Autodesk Inventor part; units mm, degrees
(part 2 of 3)
  line L384 (86.5601, -24.0434) -> (86.5601, -7.2718)
  line L385 (91.5601, -7.2718) -> (91.5601, -24.0434)
  arc A154 (86.853, -6.5647) -> (86.5601, -7.2718) centre (87.5601, -7.2718) ccw
  line L386 (86.853, -6.5647) -> (88.7601, -4.6576)
  line L387 (89.0601, -4.6576) -> (88.7601, -4.6576)
  line L388 (89.0601, -4.6576) -> (89.3601, -4.6576)
  arc A155 (91.5601, -7.2718) -> (91.2672, -6.5647) centre (90.5601, -7.2718) ccw
  line L389 (91.2672, -6.5647) -> (89.3601, -4.6576)
  arc A156 (116.0672, 0.0495) -> (116.3601, 0.7566) centre (115.3601, 0.7566) ccw
  arc A157 (111.3601, 0.7566) -> (111.653, 0.0495) centre (112.3601, 0.7566) ccw
  line L390 (116.0672, 0.0495) -> (114.1601, -1.8576)
  line L391 (111.653, 0.0495) -> (113.5601, -1.8576)
  line L392 (113.8601, -1.8576) -> (114.1601, -1.8576)
  line L393 (113.8601, -1.8576) -> (113.5601, -1.8576)
  line L394 (111.3601, 0.7566) -> (111.3601, 17.5282)
  line L395 (116.3601, 17.5282) -> (116.3601, 0.7566)
  arc A158 (111.653, 18.2353) -> (111.3601, 17.5282) centre (112.3601, 17.5282) ccw
  line L396 (111.653, 18.2353) -> (113.5601, 20.1424)
  line L397 (113.8601, 20.1424) -> (113.5601, 20.1424)
  line L398 (113.8601, 20.1424) -> (114.1601, 20.1424)
  arc A159 (116.3601, 17.5282) -> (116.0672, 18.2353) centre (115.3601, 17.5282) ccw
  line L399 (116.0672, 18.2353) -> (114.1601, 20.1424)
  arc A160 (116.0672, -24.7505) -> (116.3601, -24.0434) centre (115.3601, -24.0434) ccw
  arc A161 (111.3601, -24.0434) -> (111.653, -24.7505) centre (112.3601, -24.0434) ccw
  line L400 (116.0672, -24.7505) -> (114.1601, -26.6576)
  line L401 (111.653, -24.7505) -> (113.5601, -26.6576)
  line L402 (113.8601, -26.6576) -> (114.1601, -26.6576)
  line L403 (113.8601, -26.6576) -> (113.5601, -26.6576)
  line L404 (111.3601, -24.0434) -> (111.3601, -7.2718)
  line L405 (116.3601, -7.2718) -> (116.3601, -24.0434)
  arc A162 (111.653, -6.5647) -> (111.3601, -7.2718) centre (112.3601, -7.2718) ccw
  line L406 (111.653, -6.5647) -> (113.5601, -4.6576)
  line L407 (113.8601, -4.6576) -> (113.5601, -4.6576)
  line L408 (113.8601, -4.6576) -> (114.1601, -4.6576)
  arc A163 (116.3601, -7.2718) -> (116.0672, -6.5647) centre (115.3601, -7.2718) ccw
  line L409 (116.0672, -6.5647) -> (114.1601, -4.6576)
  arc A164 (92.3672, -30.2647) -> (93.0743, -30.5576) centre (93.0743, -29.5576) ccw
  arc A165 (93.0743, -25.5576) -> (92.3672, -25.8505) centre (93.0743, -26.5576) ccw
  line L410 (92.3672, -30.2647) -> (90.4601, -28.3576)
  line L411 (92.3672, -25.8505) -> (90.4601, -27.7576)
  line L412 (90.4601, -28.0576) -> (90.4601, -28.3576)
  line L413 (90.4601, -28.0576) -> (90.4601, -27.7576)
  line L414 (93.0743, -25.5576) -> (109.8459, -25.5576)
  line L415 (109.8459, -30.5576) -> (93.0743, -30.5576)
  arc A166 (110.553, -25.8505) -> (109.8459, -25.5576) centre (109.8459, -26.5576) ccw
  line L416 (110.553, -25.8505) -> (112.4601, -27.7576)
  line L417 (112.4601, -28.0576) -> (112.4601, -27.7576)
  line L418 (112.4601, -28.0576) -> (112.4601, -28.3576)
  arc A167 (109.8459, -30.5576) -> (110.553, -30.2647) centre (109.8459, -29.5576) ccw
  line L419 (110.553, -30.2647) -> (112.4601, -28.3576)
  line L420 (-43.8399, 8.0424) -> (-42.8399, 8.0424)
  line L421 (-42.8399, 8.0424) -> (-40.8399, 6.0424)
  line L422 (-40.8399, 6.0424) -> (-40.8399, 5.0424)
  line L423 (-40.8399, 5.0424) -> (-42.8399, 3.0424)
  line L424 (-42.8399, 3.0424) -> (-43.8399, 3.0424)
  line L425 (-43.8399, 3.0424) -> (-45.8399, 5.0424)
  line L426 (-45.8399, 5.0424) -> (-45.8399, 6.0424)
  line L427 (-45.8399, 6.0424) -> (-43.8399, 8.0424)
  line L428 (-43.8399, -11.9576) -> (-42.8399, -11.9576)
  line L429 (-42.8399, -11.9576) -> (-40.8399, -13.9576)
  line L430 (-40.8399, -13.9576) -> (-40.8399, -14.9576)
  line L431 (-40.8399, -14.9576) -> (-42.8399, -16.9576)
  line L432 (-42.8399, -16.9576) -> (-43.8399, -16.9576)
  line L433 (-43.8399, -16.9576) -> (-45.8399, -14.9576)
  line L434 (-45.8399, -14.9576) -> (-45.8399, -13.9576)
  line L435 (-45.8399, -13.9576) -> (-43.8399, -11.9576)
  line L436 (40.2601, 8.0424) -> (41.2601, 8.0424)
  line L437 (41.2601, 8.0424) -> (43.2601, 6.0424)
  line L438 (43.2601, 6.0424) -> (43.2601, 5.0424)
  line L439 (43.2601, 5.0424) -> (41.2601, 3.0424)
  line L440 (41.2601, 3.0424) -> (40.2601, 3.0424)
  line L441 (40.2601, 3.0424) -> (38.2601, 5.0424)
  line L442 (38.2601, 5.0424) -> (38.2601, 6.0424)
  line L443 (38.2601, 6.0424) -> (40.2601, 8.0424)
  line L444 (40.2601, -11.9576) -> (41.2601, -11.9576)
  line L445 (41.2601, -11.9576) -> (43.2601, -13.9576)
  line L446 (43.2601, -13.9576) -> (43.2601, -14.9576)
  line L447 (43.2601, -14.9576) -> (41.2601, -16.9576)
  line L448 (41.2601, -16.9576) -> (40.2601, -16.9576)
  line L449 (40.2601, -16.9576) -> (38.2601, -14.9576)
  line L450 (38.2601, -14.9576) -> (38.2601, -13.9576)
  line L451 (38.2601, -13.9576) -> (40.2601, -11.9576)
  arc A168 (-141.5328, -5.6647) -> (-140.8257, -5.9576) centre (-140.8257, -4.9576) ccw
  arc A169 (-140.8257, -0.9576) -> (-141.5328, -1.2505) centre (-140.8257, -1.9576) ccw
  line L452 (-141.5328, -5.6647) -> (-143.4399, -3.7576)
  line L453 (-143.4399, -3.4576) -> (-143.4399, -3.1576)
  line L454 (-143.4399, -3.4576) -> (-143.4399, -3.7576)
  line L455 (-141.5328, -1.2505) -> (-143.4399, -3.1576)
  line L456 (-140.8257, -0.9576) -> (-130.0541, -0.9576)
  line L457 (-130.0541, -5.9576) -> (-140.8257, -5.9576)
  arc A170 (-129.347, -1.2505) -> (-130.0541, -0.9576) centre (-130.0541, -1.9576) ccw
  arc A171 (-130.0541, -5.9576) -> (-129.347, -5.6647) centre (-130.0541, -4.9576) ccw
  line L458 (-129.347, -5.6647) -> (-127.4399, -3.7576)
  line L459 (-127.4399, -3.4576) -> (-127.4399, -3.7576)
  line L460 (-127.4399, -3.4576) -> (-127.4399, -3.1576)
  line L461 (-129.347, -1.2505) -> (-127.4399, -3.1576)
  arc A172 (-142.2328, -0.5505) -> (-141.9399, 0.1566) centre (-142.9399, 0.1566) ccw
  arc A173 (-146.9399, 0.1566) -> (-146.647, -0.5505) centre (-145.9399, 0.1566) ccw
  line L462 (-142.2328, -0.5505) -> (-144.1399, -2.4576)
  line L463 (-144.4399, -2.4576) -> (-144.7399, -2.4576)
  line L464 (-144.4399, -2.4576) -> (-144.1399, -2.4576)
  line L465 (-146.647, -0.5505) -> (-144.7399, -2.4576)
  line L466 (-146.9399, 0.1566) -> (-146.9399, 10.9282)
  line L467 (-141.9399, 10.9282) -> (-141.9399, 0.1566)
  arc A174 (-146.647, 11.6353) -> (-146.9399, 10.9282) centre (-145.9399, 10.9282) ccw
  arc A175 (-141.9399, 10.9282) -> (-142.2328, 11.6353) centre (-142.9399, 10.9282) ccw
  line L468 (-142.2328, 11.6353) -> (-144.1399, 13.5424)
  line L469 (-144.4399, 13.5424) -> (-144.1399, 13.5424)
  line L470 (-144.4399, 13.5424) -> (-144.7399, 13.5424)
  line L471 (-146.647, 11.6353) -> (-144.7399, 13.5424)
  arc A176 (-159.5328, -5.6647) -> (-158.8257, -5.9576) centre (-158.8257, -4.9576) ccw
  arc A177 (-158.8257, -0.9576) -> (-159.5328, -1.2505) centre (-158.8257, -1.9576) ccw
  line L472 (-159.5328, -5.6647) -> (-161.4399, -3.7576)
  line L473 (-161.4399, -3.4576) -> (-161.4399, -3.1576)
  line L474 (-161.4399, -3.4576) -> (-161.4399, -3.7576)
  line L475 (-159.5328, -1.2505) -> (-161.4399, -3.1576)
  line L476 (-158.8257, -0.9576) -> (-148.0541, -0.9576)
  line L477 (-148.0541, -5.9576) -> (-158.8257, -5.9576)
  arc A178 (-147.347, -1.2505) -> (-148.0541, -0.9576) centre (-148.0541, -1.9576) ccw
  arc A179 (-148.0541, -5.9576) -> (-147.347, -5.6647) centre (-148.0541, -4.9576) ccw
  line L478 (-147.347, -5.6647) -> (-145.4399, -3.7576)
  line L479 (-145.4399, -3.4576) -> (-145.4399, -3.7576)
  line L480 (-145.4399, -3.4576) -> (-145.4399, -3.1576)
  line L481 (-147.347, -1.2505) -> (-145.4399, -3.1576)
  arc A180 (-142.2328, -18.5505) -> (-141.9399, -17.8434) centre (-142.9399, -17.8434) ccw
  arc A181 (-146.9399, -17.8434) -> (-146.647, -18.5505) centre (-145.9399, -17.8434) ccw
  line L482 (-142.2328, -18.5505) -> (-144.1399, -20.4576)
  line L483 (-144.4399, -20.4576) -> (-144.7399, -20.4576)
  line L484 (-144.4399, -20.4576) -> (-144.1399, -20.4576)
  line L485 (-146.647, -18.5505) -> (-144.7399, -20.4576)
  line L486 (-146.9399, -17.8434) -> (-146.9399, -7.0718)
  line L487 (-141.9399, -7.0718) -> (-141.9399, -17.8434)
  arc A182 (-146.647, -6.3647) -> (-146.9399, -7.0718) centre (-145.9399, -7.0718) ccw
  arc A183 (-141.9399, -7.0718) -> (-142.2328, -6.3647) centre (-142.9399, -7.0718) ccw
  line L488 (-142.2328, -6.3647) -> (-144.1399, -4.4576)
  line L489 (-144.4399, -4.4576) -> (-144.1399, -4.4576)
  line L490 (-144.4399, -4.4576) -> (-144.7399, -4.4576)
  line L491 (-146.647, -6.3647) -> (-144.7399, -4.4576)
  arc A184 (-170.0328, 10.3353) -> (-169.3257, 10.0424) centre (-169.3257, 11.0424) ccw
  arc A185 (-169.3257, 15.0424) -> (-170.0328, 14.7495) centre (-169.3257, 14.0424) ccw
  line L492 (-170.0328, 10.3353) -> (-171.9399, 12.2424)
  line L493 (-171.9399, 12.5424) -> (-171.9399, 12.8424)
  line L494 (-171.9399, 12.5424) -> (-171.9399, 12.2424)
  line L495 (-170.0328, 14.7495) -> (-171.9399, 12.8424)
  line L496 (-169.3257, 15.0424) -> (-158.5541, 15.0424)
  line L497 (-158.5541, 10.0424) -> (-169.3257, 10.0424)
  arc A186 (-157.847, 14.7495) -> (-158.5541, 15.0424) centre (-158.5541, 14.0424) ccw
  arc A187 (-158.5541, 10.0424) -> (-157.847, 10.3353) centre (-158.5541, 11.0424) ccw
  line L498 (-157.847, 10.3353) -> (-155.9399, 12.2424)
  line L499 (-155.9399, 12.5424) -> (-155.9399, 12.2424)
  line L500 (-155.9399, 12.5424) -> (-155.9399, 12.8424)
  line L501 (-157.847, 14.7495) -> (-155.9399, 12.8424)
  arc A188 (-187.0328, 10.3353) -> (-186.3257, 10.0424) centre (-186.3257, 11.0424) ccw
  arc A189 (-186.3257, 15.0424) -> (-187.0328, 14.7495) centre (-186.3257, 14.0424) ccw
  line L502 (-187.0328, 10.3353) -> (-188.9399, 12.2424)
  line L503 (-188.9399, 12.5424) -> (-188.9399, 12.8424)
  line L504 (-188.9399, 12.5424) -> (-188.9399, 12.2424)
  line L505 (-187.0328, 14.7495) -> (-188.9399, 12.8424)
  line L506 (-186.3257, 15.0424) -> (-175.5541, 15.0424)
  line L507 (-175.5541, 10.0424) -> (-186.3257, 10.0424)
  arc A190 (-174.847, 14.7495) -> (-175.5541, 15.0424) centre (-175.5541, 14.0424) ccw
  arc A191 (-175.5541, 10.0424) -> (-174.847, 10.3353) centre (-175.5541, 11.0424) ccw
  line L508 (-174.847, 10.3353) -> (-172.9399, 12.2424)
  line L509 (-172.9399, 12.5424) -> (-172.9399, 12.2424)
  line L510 (-172.9399, 12.5424) -> (-172.9399, 12.8424)
  line L511 (-174.847, 14.7495) -> (-172.9399, 12.8424)
  arc A192 (-170.2328, -3.0647) -> (-169.9399, -2.3576) centre (-170.9399, -2.3576) ccw
  arc A193 (-174.9399, -2.3576) -> (-174.647, -3.0647) centre (-173.9399, -2.3576) ccw
  line L512 (-170.2328, -3.0647) -> (-172.1399, -4.9718)
  line L513 (-172.4399, -4.9718) -> (-172.7399, -4.9718)
  line L514 (-172.4399, -4.9718) -> (-172.1399, -4.9718)
  line L515 (-174.647, -3.0647) -> (-172.7399, -4.9718)
  line L516 (-174.9399, -2.3576) -> (-174.9399, 8.414)
  line L517 (-169.9399, 8.414) -> (-169.9399, -2.3576)
  arc A194 (-174.647, 9.1211) -> (-174.9399, 8.414) centre (-173.9399, 8.414) ccw
  arc A195 (-169.9399, 8.414) -> (-170.2328, 9.1211) centre (-170.9399, 8.414) ccw
  line L518 (-170.2328, 9.1211) -> (-172.1399, 11.0282)
  line L519 (-172.4399, 11.0282) -> (-172.1399, 11.0282)
  line L520 (-172.4399, 11.0282) -> (-172.7399, 11.0282)
  line L521 (-174.647, 9.1211) -> (-172.7399, 11.0282)
  arc A196 (-170.2328, -19.5647) -> (-169.9399, -18.8576) centre (-170.9399, -18.8576) ccw
  arc A197 (-174.9399, -18.8576) -> (-174.647, -19.5647) centre (-173.9399, -18.8576) ccw
  line L522 (-170.2328, -19.5647) -> (-172.1399, -21.4718)
  line L523 (-172.4399, -21.4718) -> (-172.7399, -21.4718)
  line L524 (-172.4399, -21.4718) -> (-172.1399, -21.4718)
  line L525 (-174.647, -19.5647) -> (-172.7399, -21.4718)
  line L526 (-174.9399, -18.8576) -> (-174.9399, -8.086)
  line L527 (-169.9399, -8.086) -> (-169.9399, -18.8576)
  arc A198 (-174.647, -7.3789) -> (-174.9399, -8.086) centre (-173.9399, -8.086) ccw
  arc A199 (-169.9399, -8.086) -> (-170.2328, -7.3789) centre (-170.9399, -8.086) ccw
  line L528 (-170.2328, -7.3789) -> (-172.1399, -5.4718)
  line L529 (-172.4399, -5.4718) -> (-172.1399, -5.4718)
  line L530 (-172.4399, -5.4718) -> (-172.7399, -5.4718)
  line L531 (-174.647, -7.3789) -> (-172.7399, -5.4718)
  point P0 (-22.4267, -1.12)
  dimension "d362" = 7.5
  dimension "d363" = 17
  dimension "d364" = 7.5
  dimension "d365" = 17
  dimension "d366" = 7.5
  dimension "d367" = 0
  dimension "d368" = 0
  dimension "d369" = 0
  dimension "d370" = 0
  dimension "d371" = 0
  dimension "d372" = 15
  dimension "d373" = 0
  dimension "d374" = 16
  dimension "d375" = 6
  dimension "d376" = 6
  dimension "d377" = 13.6
  dimension "d378" = 16
  dimension "d379" = 6
  dimension "d380" = 15
  dimension "d381" = 0
  dimension "d509" = 23
  dimension "d510" = 25
  dimension "d511" = 24.6
  dimension "d514" = 0.5
sketch "Clock Front Face Outline" plane through (0, 0, 0) normal (0, 0, 1) x (1, 0, 0)
  line L0 (-365.1075, -11.3808) -> (-85.1075, -11.3808)
  line L1 (-60.1075, -36.3808) -> (-60.1075, -56.3808)
  line L2 (-85.1075, -81.3808) -> (-365.1075, -81.3808)
  line L3 (-390.1075, -56.3808) -> (-390.1075, -36.3808)
  arc A0 (-365.1075, -11.3808) -> (-390.1075, -36.3808) centre (-365.1075, -36.3808) ccw
  arc A1 (-60.1075, -36.3808) -> (-85.1075, -11.3808) centre (-85.1075, -36.3808) ccw
  arc A2 (-85.1075, -81.3808) -> (-60.1075, -56.3808) centre (-85.1075, -56.3808) ccw
  arc A3 (-390.1075, -56.3808) -> (-365.1075, -81.3808) centre (-365.1075, -56.3808) ccw
  point P0 (0, -2.2581)
  dimension "d429" = 330
  dimension "d430" = 70
  dimension "d431" = 25
  measures "d429" distance between parallel lines of L1 L3
  measures "d430" distance between parallel lines of L2 L0
  measures "d431" radius of A0
sketch "Small Segmemt" plane through (0, 0, 0) normal (0, 0, 1) x (1, 0, 0)
  arc A0 (-247.3536, -9.433) -> (-246.6465, -9.7259) centre (-246.6465, -8.7259) ccw
  arc A1 (-246.6465, -4.7259) -> (-247.3536, -5.0187) centre (-246.6465, -5.7259) ccw
  line L0 (-247.3536, -9.433) -> (-249.2607, -7.5259)
  line L1 (-249.2607, -7.2259) -> (-249.2607, -6.9259)
  line L2 (-249.2607, -7.2259) -> (-249.2607, -7.5259)
  line L3 (-247.3536, -5.0187) -> (-249.2607, -6.9259)
  line L4 (-246.6465, -4.7259) -> (-235.875, -4.7259)
  line L5 (-235.875, -9.7259) -> (-246.6465, -9.7259)
  arc A2 (-235.1679, -5.0187) -> (-235.875, -4.7259) centre (-235.875, -5.7259) ccw
  arc A3 (-235.875, -9.7259) -> (-235.1679, -9.433) centre (-235.875, -8.7259) ccw
  line L6 (-235.1679, -9.433) -> (-233.2607, -7.5259)
  line L7 (-233.2607, -7.2259) -> (-233.2607, -7.5259)
  line L8 (-233.2607, -7.2259) -> (-233.2607, -6.9259)
  line L9 (-235.1679, -5.0187) -> (-233.2607, -6.9259)
  point P0 (-225.4266, -6.7349)
  point P1 (-247.0607, -4.7259)
  point P2 (-247.0607, -9.7259)
  point P3 (-235.4607, -4.7259)
  point P4 (-235.4607, -9.7259)
  dimension "d462" = 2.2
  dimension "d463" = 2.2
  dimension "d464" = 2.2
  dimension "d465" = 2.2
  dimension "d466" = 2.2
  dimension "d467" = 2.2
  dimension "d468" = 2.2
  dimension "d469" = 1
  dimension "d470" = 5
  dimension "d471" = 2.2
  dimension "d472" = 2.2
  dimension "d473" = 135
  dimension "d474" = 16
  dimension "d475" = 135
  dimension "d476" = 2.5
  dimension "d477" = 5
  dimension "d478" = 16
  dimension "d479" = 2.2
  dimension "d480" = 0.3
  dimension "d481" = 0.3
  dimension "d482" = 0.3
  dimension "d483" = 0.3
  measures "d462" horizontal distance of point (-247.061, -9.726) L0.end
  measures "d463" horizontal distance of L8.end point (-235.461, -4.726)
  measures "d464" horizontal distance of point (-247.061, -4.726) L1.end
  measures "d465" horizontal distance of L6.end point (-235.461, -9.726)
  measures "d466" horizontal distance of L6.end point (-235.461, -9.726)
  measures "d467" horizontal distance of point (-247.061, -4.726) L1.end
  measures "d468" horizontal distance of point (-247.061, -9.726) L0.end
  measures "d469" radius of A1
  measures "d470" distance of point (-235.461, -9.726) point (-235.461, -4.726)
  measures "d471" horizontal distance of L8.end point (-235.461, -4.726)
  measures "d472" horizontal distance of point (-235.461, -9.726) L7.start
  measures "d473" angle of L5 L6
  measures "d474" horizontal distance of L6.end L1.start
  measures "d475" angle of L4 L9
  measures "d476" vertical distance of L7.start point (-235.461, -9.726)
  measures "d477" distance between parallel lines of L5 L4
  measures "d478" distance of L1.start L7.start
  measures "d479" horizontal distance of point (-247.061, -4.726) L1.start
  measures "d480" distance of L7.start L8.end
  measures "d481" distance of L6.end L7.start
  measures "d482" distance of L1.end L1.start
  measures "d483" distance of L0.end L1.start
sketch "Sketch1" plane through (0, 0, 0) normal (0, 0, 1) x (1, 0, 0)
  line L0 (-365.1075, -11.3808) -> (-85.1075, -11.3808)
  line L1 (-60.1075, -36.3808) -> (-60.1075, -56.3808)
  line L2 (-85.1075, -81.3808) -> (-365.1075, -81.3808)
  line L3 (-390.1075, -56.3808) -> (-390.1075, -36.3808)
  arc A0 (-365.1075, -11.3808) -> (-390.1075, -36.3808) centre (-365.1075, -36.3808) ccw
  arc A1 (-60.1075, -36.3808) -> (-85.1075, -11.3808) centre (-85.1075, -36.3808) ccw
  arc A2 (-85.1075, -81.3808) -> (-60.1075, -56.3808) centre (-85.1075, -56.3808) ccw
  arc A3 (-390.1075, -56.3808) -> (-365.1075, -81.3808) centre (-365.1075, -56.3808) ccw
  point P0 (0, 0)
extrude "Extrusion1" add sketch "Sketch1" along normal blind 3
sketch "Sketch5" plane through (0, 0, 3) normal (0, 0, 1) x (1, 0, 0)
  line L0 (-85.1075, -11.3808) -> (-365.1075, -11.3808) projected
  line L1 (-365.1075, -81.3808) -> (-85.1075, -81.3808) projected
  line L2 (-390.1075, -36.3808) -> (-390.1075, -56.3808) projected
  line L3 (-60.1075, -56.3808) -> (-60.1075, -36.3808) projected
  arc A0 (-138.1004, -24.0879) -> (-137.3933, -24.3808) centre (-137.3933, -23.3808) ccw
  arc A1 (-137.3933, -19.3808) -> (-138.1004, -19.6736) centre (-137.3933, -20.3808) ccw
  line L4 (-138.1004, -24.0879) -> (-140.0075, -22.1808)
  line L5 (-138.1004, -19.6736) -> (-140.0075, -21.5808)
  line L6 (-140.0075, -21.8808) -> (-140.0075, -22.1808)
  line L7 (-140.0075, -21.8808) -> (-140.0075, -21.5808)
  line L8 (-137.3933, -19.3808) -> (-120.6217, -19.3808)
  line L9 (-120.6217, -24.3808) -> (-137.3933, -24.3808)
  arc A2 (-119.9146, -19.6736) -> (-120.6217, -19.3808) centre (-120.6217, -20.3808) ccw
  line L10 (-119.9146, -19.6736) -> (-118.0075, -21.5808)
  line L11 (-118.0075, -21.8808) -> (-118.0075, -21.5808)
  line L12 (-118.0075, -21.8808) -> (-118.0075, -22.1808)
  arc A3 (-120.6217, -24.3808) -> (-119.9146, -24.0879) centre (-120.6217, -23.3808) ccw
  line L13 (-119.9146, -24.0879) -> (-118.0075, -22.1808)
  arc A4 (-138.1004, -48.8879) -> (-137.3933, -49.1808) centre (-137.3933, -48.1808) ccw
  arc A5 (-137.3933, -44.1808) -> (-138.1004, -44.4736) centre (-137.3933, -45.1808) ccw
  line L14 (-138.1004, -48.8879) -> (-140.0075, -46.9808)
  line L15 (-138.1004, -44.4736) -> (-140.0075, -46.3808)
  line L16 (-140.0075, -46.6808) -> (-140.0075, -46.9808)
  line L17 (-140.0075, -46.6808) -> (-140.0075, -46.3808)
  line L18 (-137.3933, -44.1808) -> (-120.6217, -44.1808)
  line L19 (-120.6217, -49.1808) -> (-137.3933, -49.1808)
  arc A6 (-119.9146, -44.4736) -> (-120.6217, -44.1808) centre (-120.6217, -45.1808) ccw
  line L20 (-119.9146, -44.4736) -> (-118.0075, -46.3808)
  line L21 (-118.0075, -46.6808) -> (-118.0075, -46.3808)
  line L22 (-118.0075, -46.6808) -> (-118.0075, -46.9808)
  arc A7 (-120.6217, -49.1808) -> (-119.9146, -48.8879) centre (-120.6217, -48.1808) ccw
  line L23 (-119.9146, -48.8879) -> (-118.0075, -46.9808)
  arc A8 (-139.2004, -43.3736) -> (-138.9075, -42.6665) centre (-139.9075, -42.6665) ccw
  arc A9 (-143.9075, -42.6665) -> (-143.6146, -43.3736) centre (-142.9075, -42.6665) ccw
  line L24 (-139.2004, -43.3736) -> (-141.1075, -45.2808)
  line L25 (-143.6146, -43.3736) -> (-141.7075, -45.2808)
  line L26 (-141.4075, -45.2808) -> (-141.1075, -45.2808)
  line L27 (-141.4075, -45.2808) -> (-141.7075, -45.2808)
  line L28 (-143.9075, -42.6665) -> (-143.9075, -25.895)
  line L29 (-138.9075, -25.895) -> (-138.9075, -42.6665)
  arc A10 (-143.6146, -25.1879) -> (-143.9075, -25.895) centre (-142.9075, -25.895) ccw
  line L30 (-143.6146, -25.1879) -> (-141.7075, -23.2808)
  line L31 (-141.4075, -23.2808) -> (-141.7075, -23.2808)
  line L32 (-141.4075, -23.2808) -> (-141.1075, -23.2808)
  arc A11 (-138.9075, -25.895) -> (-139.2004, -25.1879) centre (-139.9075, -25.895) ccw
  line L33 (-139.2004, -25.1879) -> (-141.1075, -23.2808)
  arc A12 (-139.2004, -68.1736) -> (-138.9075, -67.4665) centre (-139.9075, -67.4665) ccw
  arc A13 (-143.9075, -67.4665) -> (-143.6146, -68.1736) centre (-142.9075, -67.4665) ccw
  line L34 (-139.2004, -68.1736) -> (-141.1075, -70.0808)
  line L35 (-143.6146, -68.1736) -> (-141.7075, -70.0808)
  line L36 (-141.4075, -70.0808) -> (-141.1075, -70.0808)
  line L37 (-141.4075, -70.0808) -> (-141.7075, -70.0808)
  line L38 (-143.9075, -67.4665) -> (-143.9075, -50.695)
  line L39 (-138.9075, -50.695) -> (-138.9075, -67.4665)
  arc A14 (-143.6146, -49.9879) -> (-143.9075, -50.695) centre (-142.9075, -50.695) ccw
  line L40 (-143.6146, -49.9879) -> (-141.7075, -48.0808)
  line L41 (-141.4075, -48.0808) -> (-141.7075, -48.0808)
  line L42 (-141.4075, -48.0808) -> (-141.1075, -48.0808)
  arc A15 (-138.9075, -50.695) -> (-139.2004, -49.9879) centre (-139.9075, -50.695) ccw
  line L43 (-139.2004, -49.9879) -> (-141.1075, -48.0808)
  arc A16 (-114.4004, -43.3736) -> (-114.1075, -42.6665) centre (-115.1075, -42.6665) ccw
  arc A17 (-119.1075, -42.6665) -> (-118.8146, -43.3736) centre (-118.1075, -42.6665) ccw
  line L44 (-114.4004, -43.3736) -> (-116.3075, -45.2808)
  line L45 (-118.8146, -43.3736) -> (-116.9075, -45.2808)
  line L46 (-116.6075, -45.2808) -> (-116.3075, -45.2808)
  line L47 (-116.6075, -45.2808) -> (-116.9075, -45.2808)
  line L48 (-119.1075, -42.6665) -> (-119.1075, -25.895)
  line L49 (-114.1075, -25.895) -> (-114.1075, -42.6665)
  arc A18 (-118.8146, -25.1879) -> (-119.1075, -25.895) centre (-118.1075, -25.895) ccw
  line L50 (-118.8146, -25.1879) -> (-116.9075, -23.2808)
  line L51 (-116.6075, -23.2808) -> (-116.9075, -23.2808)
  line L52 (-116.6075, -23.2808) -> (-116.3075, -23.2808)
  arc A19 (-114.1075, -25.895) -> (-114.4004, -25.1879) centre (-115.1075, -25.895) ccw
  line L53 (-114.4004, -25.1879) -> (-116.3075, -23.2808)
  arc A20 (-114.4004, -68.1736) -> (-114.1075, -67.4665) centre (-115.1075, -67.4665) ccw
  arc A21 (-119.1075, -67.4665) -> (-118.8146, -68.1736) centre (-118.1075, -67.4665) ccw
  line L54 (-114.4004, -68.1736) -> (-116.3075, -70.0808)
  line L55 (-118.8146, -68.1736) -> (-116.9075, -70.0808)
  line L56 (-116.6075, -70.0808) -> (-116.3075, -70.0808)
  line L57 (-116.6075, -70.0808) -> (-116.9075, -70.0808)
  line L58 (-119.1075, -67.4665) -> (-119.1075, -50.695)
  line L59 (-114.1075, -50.695) -> (-114.1075, -67.4665)
  arc A22 (-118.8146, -49.9879) -> (-119.1075, -50.695) centre (-118.1075, -50.695) ccw
  line L60 (-118.8146, -49.9879) -> (-116.9075, -48.0808)
  line L61 (-116.6075, -48.0808) -> (-116.9075, -48.0808)
  line L62 (-116.6075, -48.0808) -> (-116.3075, -48.0808)
  arc A23 (-114.1075, -50.695) -> (-114.4004, -49.9879) centre (-115.1075, -50.695) ccw
  line L63 (-114.4004, -49.9879) -> (-116.3075, -48.0808)
  arc A24 (-138.1004, -73.6879) -> (-137.3933, -73.9808) centre (-137.3933, -72.9808) ccw
  arc A25 (-137.3933, -68.9808) -> (-138.1004, -69.2736) centre (-137.3933, -69.9808) ccw
  line L64 (-138.1004, -73.6879) -> (-140.0075, -71.7808)
  line L65 (-138.1004, -69.2736) -> (-140.0075, -71.1808)
  line L66 (-140.0075, -71.4808) -> (-140.0075, -71.7808)
  line L67 (-140.0075, -71.4808) -> (-140.0075, -71.1808)
  line L68 (-137.3933, -68.9808) -> (-120.6217, -68.9808)
  line L69 (-120.6217, -73.9808) -> (-137.3933, -73.9808)
  arc A26 (-119.9146, -69.2736) -> (-120.6217, -68.9808) centre (-120.6217, -69.9808) ccw
  line L70 (-119.9146, -69.2736) -> (-118.0075, -71.1808)
  line L71 (-118.0075, -71.4808) -> (-118.0075, -71.1808)
  line L72 (-118.0075, -71.4808) -> (-118.0075, -71.7808)
  arc A27 (-120.6217, -73.9808) -> (-119.9146, -73.6879) centre (-120.6217, -72.9808) ccw
  line L73 (-119.9146, -73.6879) -> (-118.0075, -71.7808)
  arc A28 (-184.9004, -24.0879) -> (-184.1933, -24.3808) centre (-184.1933, -23.3808) ccw
  arc A29 (-184.1933, -19.3808) -> (-184.9004, -19.6736) centre (-184.1933, -20.3808) ccw
  line L74 (-184.9004, -24.0879) -> (-186.8075, -22.1808)
  line L75 (-184.9004, -19.6736) -> (-186.8075, -21.5808)
  line L76 (-186.8075, -21.8808) -> (-186.8075, -22.1808)
  line L77 (-186.8075, -21.8808) -> (-186.8075, -21.5808)
  line L78 (-184.1933, -19.3808) -> (-167.4217, -19.3808)
  line L79 (-167.4217, -24.3808) -> (-184.1933, -24.3808)
  arc A30 (-166.7146, -19.6736) -> (-167.4217, -19.3808) centre (-167.4217, -20.3808) ccw
  line L80 (-166.7146, -19.6736) -> (-164.8075, -21.5808)
  line L81 (-164.8075, -21.8808) -> (-164.8075, -21.5808)
  line L82 (-164.8075, -21.8808) -> (-164.8075, -22.1808)
  arc A31 (-167.4217, -24.3808) -> (-166.7146, -24.0879) centre (-167.4217, -23.3808) ccw
  line L83 (-166.7146, -24.0879) -> (-164.8075, -22.1808)
  arc A32 (-184.9004, -48.8879) -> (-184.1933, -49.1808) centre (-184.1933, -48.1808) ccw
  arc A33 (-184.1933, -44.1808) -> (-184.9004, -44.4736) centre (-184.1933, -45.1808) ccw
  line L84 (-184.9004, -48.8879) -> (-186.8075, -46.9808)
  line L85 (-184.9004, -44.4736) -> (-186.8075, -46.3808)
  line L86 (-186.8075, -46.6808) -> (-186.8075, -46.9808)
  line L87 (-186.8075, -46.6808) -> (-186.8075, -46.3808)
  line L88 (-184.1933, -44.1808) -> (-167.4217, -44.1808)
  line L89 (-167.4217, -49.1808) -> (-184.1933, -49.1808)
  arc A34 (-166.7146, -44.4736) -> (-167.4217, -44.1808) centre (-167.4217, -45.1808) ccw
  line L90 (-166.7146, -44.4736) -> (-164.8075, -46.3808)
  line L91 (-164.8075, -46.6808) -> (-164.8075, -46.3808)
  line L92 (-164.8075, -46.6808) -> (-164.8075, -46.9808)
  arc A35 (-167.4217, -49.1808) -> (-166.7146, -48.8879) centre (-167.4217, -48.1808) ccw
  line L93 (-166.7146, -48.8879) -> (-164.8075, -46.9808)
  arc A36 (-186.0004, -43.3736) -> (-185.7075, -42.6665) centre (-186.7075, -42.6665) ccw
  arc A37 (-190.7075, -42.6665) -> (-190.4146, -43.3736) centre (-189.7075, -42.6665) ccw
  line L94 (-186.0004, -43.3736) -> (-187.9075, -45.2808)
  line L95 (-190.4146, -43.3736) -> (-188.5075, -45.2808)
  line L96 (-188.2075, -45.2808) -> (-187.9075, -45.2808)
  line L97 (-188.2075, -45.2808) -> (-188.5075, -45.2808)
  line L98 (-190.7075, -42.6665) -> (-190.7075, -25.895)
  line L99 (-185.7075, -25.895) -> (-185.7075, -42.6665)
  arc A38 (-190.4146, -25.1879) -> (-190.7075, -25.895) centre (-189.7075, -25.895) ccw
  line L100 (-190.4146, -25.1879) -> (-188.5075, -23.2808)
  line L101 (-188.2075, -23.2808) -> (-188.5075, -23.2808)
  line L102 (-188.2075, -23.2808) -> (-187.9075, -23.2808)
  arc A39 (-185.7075, -25.895) -> (-186.0004, -25.1879) centre (-186.7075, -25.895) ccw
  line L103 (-186.0004, -25.1879) -> (-187.9075, -23.2808)
  arc A40 (-186.0004, -68.1736) -> (-185.7075, -67.4665) centre (-186.7075, -67.4665) ccw
  arc A41 (-190.7075, -67.4665) -> (-190.4146, -68.1736) centre (-189.7075, -67.4665) ccw
  line L104 (-186.0004, -68.1736) -> (-187.9075, -70.0808)
  line L105 (-190.4146, -68.1736) -> (-188.5075, -70.0808)
  line L106 (-188.2075, -70.0808) -> (-187.9075, -70.0808)
  line L107 (-188.2075, -70.0808) -> (-188.5075, -70.0808)
  line L108 (-190.7075, -67.4665) -> (-190.7075, -50.695)
  line L109 (-185.7075, -50.695) -> (-185.7075, -67.4665)
  arc A42 (-190.4146, -49.9879) -> (-190.7075, -50.695) centre (-189.7075, -50.695) ccw
  line L110 (-190.4146, -49.9879) -> (-188.5075, -48.0808)
  line L111 (-188.2075, -48.0808) -> (-188.5075, -48.0808)
  line L112 (-188.2075, -48.0808) -> (-187.9075, -48.0808)
  arc A43 (-185.7075, -50.695) -> (-186.0004, -49.9879) centre (-186.7075, -50.695) ccw
  line L113 (-186.0004, -49.9879) -> (-187.9075, -48.0808)
  arc A44 (-161.2004, -43.3736) -> (-160.9075, -42.6665) centre (-161.9075, -42.6665) ccw
  arc A45 (-165.9075, -42.6665) -> (-165.6146, -43.3736) centre (-164.9075, -42.6665) ccw
  line L114 (-161.2004, -43.3736) -> (-163.1075, -45.2808)
  line L115 (-165.6146, -43.3736) -> (-163.7075, -45.2808)
  line L116 (-163.4075, -45.2808) -> (-163.1075, -45.2808)
  line L117 (-163.4075, -45.2808) -> (-163.7075, -45.2808)
  line L118 (-165.9075, -42.6665) -> (-165.9075, -25.895)
  line L119 (-160.9075, -25.895) -> (-160.9075, -42.6665)
  arc A46 (-165.6146, -25.1879) -> (-165.9075, -25.895) centre (-164.9075, -25.895) ccw
  line L120 (-165.6146, -25.1879) -> (-163.7075, -23.2808)
  line L121 (-163.4075, -23.2808) -> (-163.7075, -23.2808)
  line L122 (-163.4075, -23.2808) -> (-163.1075, -23.2808)
  arc A47 (-160.9075, -25.895) -> (-161.2004, -25.1879) centre (-161.9075, -25.895) ccw
  line L123 (-161.2004, -25.1879) -> (-163.1075, -23.2808)
  arc A48 (-161.2004, -68.1736) -> (-160.9075, -67.4665) centre (-161.9075, -67.4665) ccw
  arc A49 (-165.9075, -67.4665) -> (-165.6146, -68.1736) centre (-164.9075, -67.4665) ccw
  line L124 (-161.2004, -68.1736) -> (-163.1075, -70.0808)
  line L125 (-165.6146, -68.1736) -> (-163.7075, -70.0808)
  line L126 (-163.4075, -70.0808) -> (-163.1075, -70.0808)
  line L127 (-163.4075, -70.0808) -> (-163.7075, -70.0808)
  line L128 (-165.9075, -67.4665) -> (-165.9075, -50.695)
  line L129 (-160.9075, -50.695) -> (-160.9075, -67.4665)
  arc A50 (-165.6146, -49.9879) -> (-165.9075, -50.695) centre (-164.9075, -50.695) ccw
  line L130 (-165.6146, -49.9879) -> (-163.7075, -48.0808)
  line L131 (-163.4075, -48.0808) -> (-163.7075, -48.0808)
  line L132 (-163.4075, -48.0808) -> (-163.1075, -48.0808)
  arc A51 (-160.9075, -50.695) -> (-161.2004, -49.9879) centre (-161.9075, -50.695) ccw
  line L133 (-161.2004, -49.9879) -> (-163.1075, -48.0808)
  arc A52 (-184.9004, -73.6879) -> (-184.1933, -73.9808) centre (-184.1933, -72.9808) ccw
  arc A53 (-184.1933, -68.9808) -> (-184.9004, -69.2736) centre (-184.1933, -69.9808) ccw
  line L134 (-184.9004, -73.6879) -> (-186.8075, -71.7808)
  line L135 (-184.9004, -69.2736) -> (-186.8075, -71.1808)
  line L136 (-186.8075, -71.4808) -> (-186.8075, -71.7808)
  line L137 (-186.8075, -71.4808) -> (-186.8075, -71.1808)
  line L138 (-184.1933, -68.9808) -> (-167.4217, -68.9808)
  line L139 (-167.4217, -73.9808) -> (-184.1933, -73.9808)
  arc A54 (-166.7146, -69.2736) -> (-167.4217, -68.9808) centre (-167.4217, -69.9808) ccw
  line L140 (-166.7146, -69.2736) -> (-164.8075, -71.1808)
  line L141 (-164.8075, -71.4808) -> (-164.8075, -71.1808)
  line L142 (-164.8075, -71.4808) -> (-164.8075, -71.7808)
  arc A55 (-167.4217, -73.9808) -> (-166.7146, -73.6879) centre (-167.4217, -72.9808) ccw
  line L143 (-166.7146, -73.6879) -> (-164.8075, -71.7808)
  arc A56 (-222.2004, -24.0879) -> (-221.4933, -24.3808) centre (-221.4933, -23.3808) ccw
  arc A57 (-221.4933, -19.3808) -> (-222.2004, -19.6736) centre (-221.4933, -20.3808) ccw
  line L144 (-222.2004, -24.0879) -> (-224.1075, -22.1808)
  line L145 (-222.2004, -19.6736) -> (-224.1075, -21.5808)
  line L146 (-224.1075, -21.8808) -> (-224.1075, -22.1808)
  line L147 (-224.1075, -21.8808) -> (-224.1075, -21.5808)
  line L148 (-221.4933, -19.3808) -> (-204.7217, -19.3808)
  line L149 (-204.7217, -24.3808) -> (-221.4933, -24.3808)
  arc A58 (-204.0146, -19.6736) -> (-204.7217, -19.3808) centre (-204.7217, -20.3808) ccw
  line L150 (-204.0146, -19.6736) -> (-202.1075, -21.5808)
  line L151 (-202.1075, -21.8808) -> (-202.1075, -21.5808)
  line L152 (-202.1075, -21.8808) -> (-202.1075, -22.1808)
  arc A59 (-204.7217, -24.3808) -> (-204.0146, -24.0879) centre (-204.7217, -23.3808) ccw
  line L153 (-204.0146, -24.0879) -> (-202.1075, -22.1808)
  arc A60 (-222.2004, -48.8879) -> (-221.4933, -49.1808) centre (-221.4933, -48.1808) ccw
  arc A61 (-221.4933, -44.1808) -> (-222.2004, -44.4736) centre (-221.4933, -45.1808) ccw
  line L154 (-222.2004, -48.8879) -> (-224.1075, -46.9808)
  line L155 (-222.2004, -44.4736) -> (-224.1075, -46.3808)
  line L156 (-224.1075, -46.6808) -> (-224.1075, -46.9808)
  line L157 (-224.1075, -46.6808) -> (-224.1075, -46.3808)
  line L158 (-221.4933, -44.1808) -> (-204.7217, -44.1808)
  line L159 (-204.7217, -49.1808) -> (-221.4933, -49.1808)
  arc A62 (-204.0146, -44.4736) -> (-204.7217, -44.1808) centre (-204.7217, -45.1808) ccw
  line L160 (-204.0146, -44.4736) -> (-202.1075, -46.3808)
  line L161 (-202.1075, -46.6808) -> (-202.1075, -46.3808)
  line L162 (-202.1075, -46.6808) -> (-202.1075, -46.9808)
  arc A63 (-204.7217, -49.1808) -> (-204.0146, -48.8879) centre (-204.7217, -48.1808) ccw
  line L163 (-204.0146, -48.8879) -> (-202.1075, -46.9808)
  arc A64 (-223.3004, -43.3736) -> (-223.0075, -42.6665) centre (-224.0075, -42.6665) ccw
  arc A65 (-228.0075, -42.6665) -> (-227.7146, -43.3736) centre (-227.0075, -42.6665) ccw
  line L164 (-223.3004, -43.3736) -> (-225.2075, -45.2808)
  line L165 (-227.7146, -43.3736) -> (-225.8075, -45.2808)
  line L166 (-225.5075, -45.2808) -> (-225.2075, -45.2808)
  line L167 (-225.5075, -45.2808) -> (-225.8075, -45.2808)
  line L168 (-228.0075, -42.6665) -> (-228.0075, -25.895)
  line L169 (-223.0075, -25.895) -> (-223.0075, -42.6665)
  arc A66 (-227.7146, -25.1879) -> (-228.0075, -25.895) centre (-227.0075, -25.895) ccw
  line L170 (-227.7146, -25.1879) -> (-225.8075, -23.2808)
  line L171 (-225.5075, -23.2808) -> (-225.8075, -23.2808)
  line L172 (-225.5075, -23.2808) -> (-225.2075, -23.2808)
  arc A67 (-223.0075, -25.895) -> (-223.3004, -25.1879) centre (-224.0075, -25.895) ccw
  line L173 (-223.3004, -25.1879) -> (-225.2075, -23.2808)
  arc A68 (-223.3004, -68.1736) -> (-223.0075, -67.4665) centre (-224.0075, -67.4665) ccw
  arc A69 (-228.0075, -67.4665) -> (-227.7146, -68.1736) centre (-227.0075, -67.4665) ccw
  line L174 (-223.3004, -68.1736) -> (-225.2075, -70.0808)
  line L175 (-227.7146, -68.1736) -> (-225.8075, -70.0808)
  line L176 (-225.5075, -70.0808) -> (-225.2075, -70.0808)
  line L177 (-225.5075, -70.0808) -> (-225.8075, -70.0808)
  line L178 (-228.0075, -67.4665) -> (-228.0075, -50.695)
  line L179 (-223.0075, -50.695) -> (-223.0075, -67.4665)
  arc A70 (-227.7146, -49.9879) -> (-228.0075, -50.695) centre (-227.0075, -50.695) ccw
  line L180 (-227.7146, -49.9879) -> (-225.8075, -48.0808)
  line L181 (-225.5075, -48.0808) -> (-225.8075, -48.0808)
  line L182 (-225.5075, -48.0808) -> (-225.2075, -48.0808)
  arc A71 (-223.0075, -50.695) -> (-223.3004, -49.9879) centre (-224.0075, -50.695) ccw
  line L183 (-223.3004, -49.9879) -> (-225.2075, -48.0808)
  arc A72 (-198.5004, -43.3736) -> (-198.2075, -42.6665) centre (-199.2075, -42.6665) ccw
  arc A73 (-203.2075, -42.6665) -> (-202.9146, -43.3736) centre (-202.2075, -42.6665) ccw
  line L184 (-198.5004, -43.3736) -> (-200.4075, -45.2808)
  line L185 (-202.9146, -43.3736) -> (-201.0075, -45.2808)
  line L186 (-200.7075, -45.2808) -> (-200.4075, -45.2808)
  line L187 (-200.7075, -45.2808) -> (-201.0075, -45.2808)
  line L188 (-203.2075, -42.6665) -> (-203.2075, -25.895)
  line L189 (-198.2075, -25.895) -> (-198.2075, -42.6665)
  arc A74 (-202.9146, -25.1879) -> (-203.2075, -25.895) centre (-202.2075, -25.895) ccw
  line L190 (-202.9146, -25.1879) -> (-201.0075, -23.2808)
  line L191 (-200.7075, -23.2808) -> (-201.0075, -23.2808)
  line L192 (-200.7075, -23.2808) -> (-200.4075, -23.2808)
  arc A75 (-198.2075, -25.895) -> (-198.5004, -25.1879) centre (-199.2075, -25.895) ccw
  line L193 (-198.5004, -25.1879) -> (-200.4075, -23.2808)
  arc A76 (-198.5004, -68.1736) -> (-198.2075, -67.4665) centre (-199.2075, -67.4665) ccw
  arc A77 (-203.2075, -67.4665) -> (-202.9146, -68.1736) centre (-202.2075, -67.4665) ccw
  line L194 (-198.5004, -68.1736) -> (-200.4075, -70.0808)
  line L195 (-202.9146, -68.1736) -> (-201.0075, -70.0808)
  line L196 (-200.7075, -70.0808) -> (-200.4075, -70.0808)
  line L197 (-200.7075, -70.0808) -> (-201.0075, -70.0808)
  line L198 (-203.2075, -67.4665) -> (-203.2075, -50.695)
  line L199 (-198.2075, -50.695) -> (-198.2075, -67.4665)
  arc A78 (-202.9146, -49.9879) -> (-203.2075, -50.695) centre (-202.2075, -50.695) ccw
  line L200 (-202.9146, -49.9879) -> (-201.0075, -48.0808)
  line L201 (-200.7075, -48.0808) -> (-201.0075, -48.0808)
  line L202 (-200.7075, -48.0808) -> (-200.4075, -48.0808)
  arc A79 (-198.2075, -50.695) -> (-198.5004, -49.9879) centre (-199.2075, -50.695) ccw
  line L203 (-198.5004, -49.9879) -> (-200.4075, -48.0808)
  arc A80 (-222.2004, -73.6879) -> (-221.4933, -73.9808) centre (-221.4933, -72.9808) ccw
  arc A81 (-221.4933, -68.9808) -> (-222.2004, -69.2736) centre (-221.4933, -69.9808) ccw
  line L204 (-222.2004, -73.6879) -> (-224.1075, -71.7808)
  line L205 (-222.2004, -69.2736) -> (-224.1075, -71.1808)
  line L206 (-224.1075, -71.4808) -> (-224.1075, -71.7808)
  line L207 (-224.1075, -71.4808) -> (-224.1075, -71.1808)
  line L208 (-221.4933, -68.9808) -> (-204.7217, -68.9808)
  line L209 (-204.7217, -73.9808) -> (-221.4933, -73.9808)
  arc A82 (-204.0146, -69.2736) -> (-204.7217, -68.9808) centre (-204.7217, -69.9808) ccw
  line L210 (-204.0146, -69.2736) -> (-202.1075, -71.1808)
  line L211 (-202.1075, -71.4808) -> (-202.1075, -71.1808)
  line L212 (-202.1075, -71.4808) -> (-202.1075, -71.7808)
  arc A83 (-204.7217, -73.9808) -> (-204.0146, -73.6879) centre (-204.7217, -72.9808) ccw
  line L213 (-204.0146, -73.6879) -> (-202.1075, -71.7808)
  arc A84 (-269.0004, -24.0879) -> (-268.2933, -24.3808) centre (-268.2933, -23.3808) ccw
  arc A85 (-268.2933, -19.3808) -> (-269.0004, -19.6736) centre (-268.2933, -20.3808) ccw
  line L214 (-269.0004, -24.0879) -> (-270.9075, -22.1808)
  line L215 (-269.0004, -19.6736) -> (-270.9075, -21.5808)
  line L216 (-270.9075, -21.8808) -> (-270.9075, -22.1808)
  line L217 (-270.9075, -21.8808) -> (-270.9075, -21.5808)
  line L218 (-268.2933, -19.3808) -> (-251.5217, -19.3808)
  line L219 (-251.5217, -24.3808) -> (-268.2933, -24.3808)
  arc A86 (-250.8146, -19.6736) -> (-251.5217, -19.3808) centre (-251.5217, -20.3808) ccw
  line L220 (-250.8146, -19.6736) -> (-248.9075, -21.5808)
  line L221 (-248.9075, -21.8808) -> (-248.9075, -21.5808)
  line L222 (-248.9075, -21.8808) -> (-248.9075, -22.1808)
  arc A87 (-251.5217, -24.3808) -> (-250.8146, -24.0879) centre (-251.5217, -23.3808) ccw
  line L223 (-250.8146, -24.0879) -> (-248.9075, -22.1808)
  arc A88 (-269.0004, -48.8879) -> (-268.2933, -49.1808) centre (-268.2933, -48.1808) ccw
  arc A89 (-268.2933, -44.1808) -> (-269.0004, -44.4736) centre (-268.2933, -45.1808) ccw
  line L224 (-269.0004, -48.8879) -> (-270.9075, -46.9808)
  line L225 (-269.0004, -44.4736) -> (-270.9075, -46.3808)
  line L226 (-270.9075, -46.6808) -> (-270.9075, -46.9808)
  line L227 (-270.9075, -46.6808) -> (-270.9075, -46.3808)
  line L228 (-268.2933, -44.1808) -> (-251.5217, -44.1808)
  line L229 (-251.5217, -49.1808) -> (-268.2933, -49.1808)
  arc A90 (-250.8146, -44.4736) -> (-251.5217, -44.1808) centre (-251.5217, -45.1808) ccw
  line L230 (-250.8146, -44.4736) -> (-248.9075, -46.3808)
  line L231 (-248.9075, -46.6808) -> (-248.9075, -46.3808)
  line L232 (-248.9075, -46.6808) -> (-248.9075, -46.9808)
  arc A91 (-251.5217, -49.1808) -> (-250.8146, -48.8879) centre (-251.5217, -48.1808) ccw
  line L233 (-250.8146, -48.8879) -> (-248.9075, -46.9808)
  arc A92 (-270.1004, -43.3736) -> (-269.8075, -42.6665) centre (-270.8075, -42.6665) ccw
  arc A93 (-274.8075, -42.6665) -> (-274.5146, -43.3736) centre (-273.8075, -42.6665) ccw
  line L234 (-270.1004, -43.3736) -> (-272.0075, -45.2808)
  line L235 (-274.5146, -43.3736) -> (-272.6075, -45.2808)
  line L236 (-272.3075, -45.2808) -> (-272.0075, -45.2808)
  line L237 (-272.3075, -45.2808) -> (-272.6075, -45.2808)
  line L238 (-274.8075, -42.6665) -> (-274.8075, -25.895)
  line L239 (-269.8075, -25.895) -> (-269.8075, -42.6665)
  arc A94 (-274.5146, -25.1879) -> (-274.8075, -25.895) centre (-273.8075, -25.895) ccw
  line L240 (-274.5146, -25.1879) -> (-272.6075, -23.2808)
  line L241 (-272.3075, -23.2808) -> (-272.6075, -23.2808)
  line L242 (-272.3075, -23.2808) -> (-272.0075, -23.2808)
  arc A95 (-269.8075, -25.895) -> (-270.1004, -25.1879) centre (-270.8075, -25.895) ccw
  line L243 (-270.1004, -25.1879) -> (-272.0075, -23.2808)
  arc A96 (-270.1004, -68.1736) -> (-269.8075, -67.4665) centre (-270.8075, -67.4665) ccw
  arc A97 (-274.8075, -67.4665) -> (-274.5146, -68.1736) centre (-273.8075, -67.4665) ccw
  line L244 (-270.1004, -68.1736) -> (-272.0075, -70.0808)
  line L245 (-274.5146, -68.1736) -> (-272.6075, -70.0808)
  line L246 (-272.3075, -70.0808) -> (-272.0075, -70.0808)
  line L247 (-272.3075, -70.0808) -> (-272.6075, -70.0808)
  line L248 (-274.8075, -67.4665) -> (-274.8075, -50.695)
  line L249 (-269.8075, -50.695) -> (-269.8075, -67.4665)
  arc A98 (-274.5146, -49.9879) -> (-274.8075, -50.695) centre (-273.8075, -50.695) ccw
  line L250 (-274.5146, -49.9879) -> (-272.6075, -48.0808)
  line L251 (-272.3075, -48.0808) -> (-272.6075, -48.0808)
  line L252 (-272.3075, -48.0808) -> (-272.0075, -48.0808)
  arc A99 (-269.8075, -50.695) -> (-270.1004, -49.9879) centre (-270.8075, -50.695) ccw
  line L253 (-270.1004, -49.9879) -> (-272.0075, -48.0808)
  arc A100 (-245.3004, -43.3736) -> (-245.0075, -42.6665) centre (-246.0075, -42.6665) ccw
  arc A101 (-250.0075, -42.6665) -> (-249.7146, -43.3736) centre (-249.0075, -42.6665) ccw
  line L254 (-245.3004, -43.3736) -> (-247.2075, -45.2808)
  line L255 (-249.7146, -43.3736) -> (-247.8075, -45.2808)
  line L256 (-247.5075, -45.2808) -> (-247.2075, -45.2808)
  line L257 (-247.5075, -45.2808) -> (-247.8075, -45.2808)
  line L258 (-250.0075, -42.6665) -> (-250.0075, -25.895)
  line L259 (-245.0075, -25.895) -> (-245.0075, -42.6665)
  arc A102 (-249.7146, -25.1879) -> (-250.0075, -25.895) centre (-249.0075, -25.895) ccw
  line L260 (-249.7146, -25.1879) -> (-247.8075, -23.2808)
  line L261 (-247.5075, -23.2808) -> (-247.8075, -23.2808)
  line L262 (-247.5075, -23.2808) -> (-247.2075, -23.2808)
  arc A103 (-245.0075, -25.895) -> (-245.3004, -25.1879) centre (-246.0075, -25.895) ccw
  line L263 (-245.3004, -25.1879) -> (-247.2075, -23.2808)
  arc A104 (-245.3004, -68.1736) -> (-245.0075, -67.4665) centre (-246.0075, -67.4665) ccw
  arc A105 (-250.0075, -67.4665) -> (-249.7146, -68.1736) centre (-249.0075, -67.4665) ccw
  line L264 (-245.3004, -68.1736) -> (-247.2075, -70.0808)
  line L265 (-249.7146, -68.1736) -> (-247.8075, -70.0808)
  line L266 (-247.5075, -70.0808) -> (-247.2075, -70.0808)
  line L267 (-247.5075, -70.0808) -> (-247.8075, -70.0808)
  line L268 (-250.0075, -67.4665) -> (-250.0075, -50.695)
  line L269 (-245.0075, -50.695) -> (-245.0075, -67.4665)
  arc A106 (-249.7146, -49.9879) -> (-250.0075, -50.695) centre (-249.0075, -50.695) ccw
  line L270 (-249.7146, -49.9879) -> (-247.8075, -48.0808)
  line L271 (-247.5075, -48.0808) -> (-247.8075, -48.0808)
  line L272 (-247.5075, -48.0808) -> (-247.2075, -48.0808)
  arc A107 (-245.0075, -50.695) -> (-245.3004, -49.9879) centre (-246.0075, -50.695) ccw
  line L273 (-245.3004, -49.9879) -> (-247.2075, -48.0808)
  arc A108 (-269.0004, -73.6879) -> (-268.2933, -73.9808) centre (-268.2933, -72.9808) ccw
  arc A109 (-268.2933, -68.9808) -> (-269.0004, -69.2736) centre (-268.2933, -69.9808) ccw
  line L274 (-269.0004, -73.6879) -> (-270.9075, -71.7808)
  line L275 (-269.0004, -69.2736) -> (-270.9075, -71.1808)
  line L276 (-270.9075, -71.4808) -> (-270.9075, -71.7808)
  line L277 (-270.9075, -71.4808) -> (-270.9075, -71.1808)
  line L278 (-268.2933, -68.9808) -> (-251.5217, -68.9808)
  line L279 (-251.5217, -73.9808) -> (-268.2933, -73.9808)
  arc A110 (-250.8146, -69.2736) -> (-251.5217, -68.9808) centre (-251.5217, -69.9808) ccw
  line L280 (-250.8146, -69.2736) -> (-248.9075, -71.1808)
  line L281 (-248.9075, -71.4808) -> (-248.9075, -71.1808)
  line L282 (-248.9075, -71.4808) -> (-248.9075, -71.7808)
  arc A111 (-251.5217, -73.9808) -> (-250.8146, -73.6879) centre (-251.5217, -72.9808) ccw
  line L283 (-250.8146, -73.6879) -> (-248.9075, -71.7808)
  arc A112 (-306.3004, -24.0879) -> (-305.5933, -24.3808) centre (-305.5933, -23.3808) ccw
  arc A113 (-305.5933, -19.3808) -> (-306.3004, -19.6736) centre (-305.5933, -20.3808) ccw
  line L284 (-306.3004, -24.0879) -> (-308.2075, -22.1808)
  line L285 (-306.3004, -19.6736) -> (-308.2075, -21.5808)
  line L286 (-308.2075, -21.8808) -> (-308.2075, -22.1808)
  line L287 (-308.2075, -21.8808) -> (-308.2075, -21.5808)
  line L288 (-305.5933, -19.3808) -> (-288.8217, -19.3808)
  line L289 (-288.8217, -24.3808) -> (-305.5933, -24.3808)
  arc A114 (-288.1146, -19.6736) -> (-288.8217, -19.3808) centre (-288.8217, -20.3808) ccw
  line L290 (-288.1146, -19.6736) -> (-286.2075, -21.5808)
  line L291 (-286.2075, -21.8808) -> (-286.2075, -21.5808)
  line L292 (-286.2075, -21.8808) -> (-286.2075, -22.1808)
  arc A115 (-288.8217, -24.3808) -> (-288.1146, -24.0879) centre (-288.8217, -23.3808) ccw
  line L293 (-288.1146, -24.0879) -> (-286.2075, -22.1808)
  arc A116 (-306.3004, -48.8879) -> (-305.5933, -49.1808) centre (-305.5933, -48.1808) ccw
  arc A117 (-305.5933, -44.1808) -> (-306.3004, -44.4736) centre (-305.5933, -45.1808) ccw
  line L294 (-306.3004, -48.8879) -> (-308.2075, -46.9808)
  line L295 (-306.3004, -44.4736) -> (-308.2075, -46.3808)
  line L296 (-308.2075, -46.6808) -> (-308.2075, -46.9808)
  line L297 (-308.2075, -46.6808) -> (-308.2075, -46.3808)
  line L298 (-305.5933, -44.1808) -> (-288.8217, -44.1808)
  line L299 (-288.8217, -49.1808) -> (-305.5933, -49.1808)
  arc A118 (-288.1146, -44.4736) -> (-288.8217, -44.1808) centre (-288.8217, -45.1808) ccw
  line L300 (-288.1146, -44.4736) -> (-286.2075, -46.3808)
  line L301 (-286.2075, -46.6808) -> (-286.2075, -46.3808)
  line L302 (-286.2075, -46.6808) -> (-286.2075, -46.9808)
  arc A119 (-288.8217, -49.1808) -> (-288.1146, -48.8879) centre (-288.8217, -48.1808) ccw
  line L303 (-288.1146, -48.8879) -> (-286.2075, -46.9808)
  arc A120 (-307.4004, -43.3736) -> (-307.1075, -42.6665) centre (-308.1075, -42.6665) ccw
  arc A121 (-312.1075, -42.6665) -> (-311.8146, -43.3736) centre (-311.1075, -42.6665) ccw
  line L304 (-307.4004, -43.3736) -> (-309.3075, -45.2808)
  line L305 (-311.8146, -43.3736) -> (-309.9075, -45.2808)
  line L306 (-309.6075, -45.2808) -> (-309.3075, -45.2808)
  line L307 (-309.6075, -45.2808) -> (-309.9075, -45.2808)
  line L308 (-312.1075, -42.6665) -> (-312.1075, -25.895)
  line L309 (-307.1075, -25.895) -> (-307.1075, -42.6665)
  arc A122 (-311.8146, -25.1879) -> (-312.1075, -25.895) centre (-311.1075, -25.895) ccw
  line L310 (-311.8146, -25.1879) -> (-309.9075, -23.2808)
  line L311 (-309.6075, -23.2808) -> (-309.9075, -23.2808)
  line L312 (-309.6075, -23.2808) -> (-309.3075, -23.2808)
  arc A123 (-307.1075, -25.895) -> (-307.4004, -25.1879) centre (-308.1075, -25.895) ccw
  line L313 (-307.4004, -25.1879) -> (-309.3075, -23.2808)
  arc A124 (-307.4004, -68.1736) -> (-307.1075, -67.4665) centre (-308.1075, -67.4665) ccw
  arc A125 (-312.1075, -67.4665) -> (-311.8146, -68.1736) centre (-311.1075, -67.4665) ccw
  line L314 (-307.4004, -68.1736) -> (-309.3075, -70.0808)
  line L315 (-311.8146, -68.1736) -> (-309.9075, -70.0808)
  line L316 (-309.6075, -70.0808) -> (-309.3075, -70.0808)
  line L317 (-309.6075, -70.0808) -> (-309.9075, -70.0808)
  line L318 (-312.1075, -67.4665) -> (-312.1075, -50.695)
  line L319 (-307.1075, -50.695) -> (-307.1075, -67.4665)
  arc A126 (-311.8146, -49.9879) -> (-312.1075, -50.695) centre (-311.1075, -50.695) ccw
  line L320 (-311.8146, -49.9879) -> (-309.9075, -48.0808)
  line L321 (-309.6075, -48.0808) -> (-309.9075, -48.0808)
  line L322 (-309.6075, -48.0808) -> (-309.3075, -48.0808)
  arc A127 (-307.1075, -50.695) -> (-307.4004, -49.9879) centre (-308.1075, -50.695) ccw
  line L323 (-307.4004, -49.9879) -> (-309.3075, -48.0808)
  arc A128 (-282.6004, -43.3736) -> (-282.3075, -42.6665) centre (-283.3075, -42.6665) ccw
  arc A129 (-287.3075, -42.6665) -> (-287.0146, -43.3736) centre (-286.3075, -42.6665) ccw
  line L324 (-282.6004, -43.3736) -> (-284.5075, -45.2808)
  line L325 (-287.0146, -43.3736) -> (-285.1075, -45.2808)
  line L326 (-284.8075, -45.2808) -> (-284.5075, -45.2808)
  line L327 (-284.8075, -45.2808) -> (-285.1075, -45.2808)
  line L328 (-287.3075, -42.6665) -> (-287.3075, -25.895)
  line L329 (-282.3075, -25.895) -> (-282.3075, -42.6665)
  arc A130 (-287.0146, -25.1879) -> (-287.3075, -25.895) centre (-286.3075, -25.895) ccw
  line L330 (-287.0146, -25.1879) -> (-285.1075, -23.2808)
  line L331 (-284.8075, -23.2808) -> (-285.1075, -23.2808)
  line L332 (-284.8075, -23.2808) -> (-284.5075, -23.2808)
  arc A131 (-282.3075, -25.895) -> (-282.6004, -25.1879) centre (-283.3075, -25.895) ccw
  line L333 (-282.6004, -25.1879) -> (-284.5075, -23.2808)
  arc A132 (-282.6004, -68.1736) -> (-282.3075, -67.4665) centre (-283.3075, -67.4665) ccw
  arc A133 (-287.3075, -67.4665) -> (-287.0146, -68.1736) centre (-286.3075, -67.4665) ccw
  line L334 (-282.6004, -68.1736) -> (-284.5075, -70.0808)
  line L335 (-287.0146, -68.1736) -> (-285.1075, -70.0808)
  line L336 (-284.8075, -70.0808) -> (-284.5075, -70.0808)
  line L337 (-284.8075, -70.0808) -> (-285.1075, -70.0808)
  line L338 (-287.3075, -67.4665) -> (-287.3075, -50.695)
  line L339 (-282.3075, -50.695) -> (-282.3075, -67.4665)
  arc A134 (-287.0146, -49.9879) -> (-287.3075, -50.695) centre (-286.3075, -50.695) ccw
  line L340 (-287.0146, -49.9879) -> (-285.1075, -48.0808)
  line L341 (-284.8075, -48.0808) -> (-285.1075, -48.0808)
  line L342 (-284.8075, -48.0808) -> (-284.5075, -48.0808)
  arc A135 (-282.3075, -50.695) -> (-282.6004, -49.9879) centre (-283.3075, -50.695) ccw
  line L343 (-282.6004, -49.9879) -> (-284.5075, -48.0808)